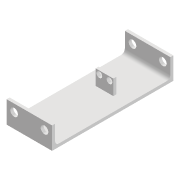
# Autodesk Inventor part: Top grip collecter grip
Saved by Autodesk Inventor 2020 (Build 240168000, 168)
## iProperties
Created: 2019-10-17
Part Number: Top grip collecter grip
Material: Generic
Document SubType Name: Modeling
Designer: ball
Density: 1 g/cm^3
Appearance: Default
Author: ball
Autodesk Inventor part; units mm, degrees
ref_plane "YZ Plane" through (0, 0, 0) normal (1, 0, 0) x (0, 1, 0)
ref_plane "XZ Plane" through (0, 0, 0) normal (0, 1, 0) x (-1, 0, 0)
sketch "Sketch1" plane through (0, 0, 0) normal (0, 1, 0) x (-1, 0, 0)
  line L0 (0, 0) -> (76.2, 0)
  line L1 (76.2, 0) -> (76.2, -203.2)
  line L2 (76.2, -203.2) -> (0, -203.2)
  line L3 (0, -203.2) -> (0, 0)
  dimension "d0" = 76.2
  dimension "d1" = 203.2
  constraints: 8 end point, 2 parallel, 1 horizontal, 1 perpendicular
  measures "d0" distance of L1.end L2.end
  measures "d1" distance of L0.end L1.end
extrude "Extrusion1" add sketch "Sketch1" along normal blind 36.83
sketch "Sketch2" plane through (-76.2, 0, 0) normal (0, 0, 1) x (1, 0, 0)
  circle A0 centre (63.5, 24.13) radius 6.4135
  circle A1 centre (12.7, 24.13) radius 6.4135
  line L0 (76.2, 0) -> (0, 0) projected
  line L1 (0, 0) -> (0, 36.83) projected
  dimension "d4" = 12.827
  dimension "d5" = 12.827
  dimension "d6" = 24.13
  dimension "d7" = 24.13
  dimension "d8" = 50.8
  dimension "d9" = 12.7
  constraints: 2 centre point
  measures "d4" diameter of A0
  measures "d5" diameter of A1
  measures "d6" distance from line of L0 A1.centre
  measures "d7" distance from line of L0 A0.centre
  measures "d8" distance of A0.centre A1.centre
  measures "d9" distance from line of L1 A1.centre
extrude "Extrusion2" cut sketch "Sketch2" against normal through all
sketch "Sketch3" plane through (0, 0, 0) normal (1, 0, 0) x (0, 0, -1)
  line L0 (0, 36.83) -> (203.2, 36.83) projected
  line L1 (5.08, 36.83) -> (198.12, 36.83)
  line L2 (198.12, 36.83) -> (198.12, 5.08)
  line L3 (198.12, 5.08) -> (5.08, 5.08)
  line L4 (5.08, 5.08) -> (5.08, 36.83)
  line L5 (0, 0) -> (0, 36.83) projected
  line L6 (203.2, 0) -> (203.2, 36.83) projected
  line L7 (203.2, 0) -> (0, 0) projected
  dimension "d12" = 5.08
  dimension "d13" = 5.08
  dimension "d14" = 5.08
  constraints: 8 end point, 2 parallel, 1 horizontal, 1 perpendicular, 1 point on line
  measures "d12" distance between parallel lines of L5 L4
  measures "d13" distance between parallel lines of L6 L2
  measures "d14" distance between parallel lines of L7 L3
extrude "Extrusion3" cut sketch "Sketch3" against normal through all contours L0 L2 L3 L4
fillet "Fillet1" radius 6.35 2 edges at (-38.1, 5.08, -198.12) (-38.1, 5.08, -5.08)
ref_plane "Work Plane1" through (-38.1, 0, 0) normal (1, 0, 0) x (0, 0, -1)
sketch "Sketch4" plane through (0, 5.08, -11.43) normal (0, 1, 0) x (1, 0, 0)
  line L0 (-60.3288, -11.303) -> (-60.3288, 191.643) construction
  line L1 (-15.4638, -11.303) -> (-15.4638, 191.643) construction
  line L2 (-23.0838, 119.2895) -> (-52.7088, 119.2895)
  line L3 (-52.7088, 114.2095) -> (-23.0838, 114.2095)
  line L4 (-52.7088, 114.2095) -> (-52.7088, 119.2895)
  line L5 (-23.0838, 114.2095) -> (-23.0838, 119.2895)
  line L6 (-24.257, 119.5032) -> (-34.9758, 119.5032) projected
  point P0 (0, -11.43)
  dimension "d19" = 7.62
  dimension "d20" = 7.62
  constraints: 10 end point, 2 perpendicular, 1 horizontal, 1 parallel, 1 vertical, 2 other
  measures "d19" distance between parallel lines of L0 L4
  measures "d20" distance between parallel lines of L1 L5
extrude "Extrusion4" add sketch "Sketch4" along normal blind 25.4
sketch "Sketch7" plane through (-52.7088, 5.08, -125.6395) normal (0, 0, 1) x (1, 0, 0)
  circle A0 centre (6.1541, 19.4644) radius 5.0173 construction
  circle A1 centre (6.1541, 19.4644) radius 4.826
  circle A2 centre (23.0924, 19.1199) radius 4.826
  circle A3 centre (23.0924, 19.462) radius 5.3594 projected
  circle A4 centre (6.1541, 19.8066) radius 5.3594 projected
  point P0 (52.7088, -5.08)
  dimension "d23" = 9.652
  dimension "d24" = 9.652
  constraints: 3 centre point, 1 coincident, 1 tangent
  measures "d23" diameter of A1
  measures "d24" diameter of A2
extrude "Extrusion5" cut sketch "Sketch7" against normal blind 6.35 contours A1 | A2
fillet "Fillet2" radius 3.175 4 edges at (-37.8963, 5.08, -125.6395) (-37.8963, 5.08, -130.7195) (-23.0838, 5.08, -128.1795) (-52.7088, 5.08, -128.1795)
sketch "Sketch8" plane through (0, 5.08, -11.43) normal (0, 1, 0) x (1, 0, 0)
  line L0 (-25.9664, 160.17) -> (-33.2664, 160.17) construction
  line L1 (-15.4638, -11.303) -> (-15.4638, 191.643) construction
  ellipse E0 centre (-46.5547, 158.3808) end of major axis (-51.9141, 158.3808) minor radius 0.1316 construction
  ellipse E1 centre (-46.5547, 161.5041) end of major axis (-51.3045, 161.5041) minor radius 0.1166 construction
  line L2 (-60.3288, -11.303) -> (-60.3288, 191.643) construction
  line L3 (-60.3288, -11.303) -> (-60.3288, 191.643) construction
  line L4 (-19.7164, 160.04) -> (-19.541, 180.14) construction
  line L5 (-19.7164, 160.04) -> (-19.541, 180.14) construction
  line L6 (-19.6387, 168.9455) -> (-19.673, 165.0128) construction
  line L7 (-19.6387, 168.9455) -> (-19.6387, 168.9455) construction
  line L8 (-19.6283, 170.1318) -> (-19.6387, 168.9455) construction
  line L9 (-19.6283, 170.1318) -> (-19.6283, 170.1318) construction
  line L10 (-19.6283, 170.1336) -> (-19.6283, 170.1318) construction
  line L11 (-19.6094, 172.2957) -> (-19.6283, 170.1336) construction
  line L12 (-19.6094, 172.2984) -> (-19.6094, 172.2957) construction
  line L13 (-19.6094, 172.2957) -> (-19.6094, 172.2984) construction
  line L14 (-19.6515, 167.4818) -> (-19.6094, 172.2957) construction
  line L15 (-19.6528, 167.3259) -> (-19.6515, 167.4818) construction
  line L16 (-19.6528, 167.3259) -> (-19.6528, 167.3259) construction
  line L17 (-19.6679, 165.5962) -> (-19.6528, 167.3259) construction
  line L18 (-19.6679, 165.5962) -> (-19.6679, 165.5962) construction
  line L19 (-19.653, 167.3096) -> (-19.6679, 165.5962) construction
  line L20 (-19.653, 167.3096) -> (-19.6494, 167.7197) construction
  line L21 (-19.6094, 172.2957) -> (-19.6494, 167.7197) construction
  line L22 (-19.6283, 170.1318) -> (-19.6094, 172.2957) construction
  line L23 (-19.6283, 170.1318) -> (-19.6283, 170.1318) construction
  line L24 (-19.6283, 170.13) -> (-19.6283, 170.1318) construction
  line L25 (-19.6717, 165.1614) -> (-19.6283, 170.13) construction
  line L26 (-19.6868, 163.4314) -> (-19.6717, 165.1614) construction
  line L27 (-19.6868, 163.4314) -> (-19.6868, 163.4314) construction
  line L28 (-19.673, 165.0128) -> (-19.6868, 163.4314) construction
  line L29 (-19.6094, 172.2957) -> (-19.6283, 170.1318) construction
  line L30 (-19.6094, 172.2957) -> (-19.6094, 172.2957) construction
  line L31 (-19.673, 165.0128) -> (-19.6094, 172.2957) construction
  line L32 (-19.6868, 163.4314) -> (-19.673, 165.0128) construction
  line L33 (-19.6868, 163.4314) -> (-19.6868, 163.4314) construction
  line L34 (-19.6868, 163.4334) -> (-19.6868, 163.4314) construction
  line L35 (-19.6679, 165.5962) -> (-19.6868, 163.4334) construction
  line L36 (-19.6679, 165.5962) -> (-19.6679, 165.5962) construction
  line L37 (-19.6679, 165.5979) -> (-19.6679, 165.5962) construction
  line L38 (-19.6552, 167.0544) -> (-19.6679, 165.5979) construction
  line L39 (-19.6552, 167.0544) -> (-19.6552, 167.0544) construction
  line L40 (-19.6411, 168.6735) -> (-19.6552, 167.0544) construction
  line L41 (-19.6411, 168.6735) -> (-19.6411, 168.6735) construction
  line L42 (-19.6283, 170.1318) -> (-19.6411, 168.6735) construction
  line L43 (-19.6283, 170.1318) -> (-19.6283, 170.1318) construction
  line L44 (-19.6868, 163.4314) -> (-19.6868, 163.4314) construction
  line L45 (-19.6094, 172.2957) -> (-19.6868, 163.4314) construction
  line L46 (-19.6868, 163.4314) -> (-19.6094, 172.2957) construction
  line L47 (-19.6868, 163.4314) -> (-19.6868, 163.4314) construction
  line L48 (-19.6472, 167.967) -> (-19.6868, 163.4314) construction
  line L49 (-19.6868, 163.4314) -> (-19.6472, 167.967) construction
  line L50 (-19.5888, 174.6572) -> (-19.584, 175.214) construction
  line L51 (-19.5788, 175.8099) -> (-19.5739, 176.3668) construction
  line L52 (-19.5858, 175.0075) -> (-19.5736, 176.4035) construction
  line L53 (-19.5736, 176.4035) -> (-19.5736, 176.4035) construction
  line L54 (-19.5736, 176.4035) -> (-19.5858, 175.0075) construction
  line L55 (-19.5858, 175.0075) -> (-19.5858, 175.0075) construction
  line L56 (-19.5858, 175.0075) -> (-19.5892, 174.6137) construction
  line L57 (-19.5892, 174.6137) -> (-19.5892, 174.6137) construction
  line L58 (-19.5892, 174.6137) -> (-19.5858, 175.0075) construction
  line L59 (-19.5858, 175.0075) -> (-19.5858, 175.0075) construction
  line L60 (-19.5844, 175.1679) -> (-19.5884, 174.7078) construction
  line L61 (-19.5831, 175.3099) -> (-19.5834, 175.2759) construction
  line L62 (-19.5789, 175.7906) -> (-19.5747, 176.2825) construction
  line L63 (-19.5781, 175.8923) -> (-19.5789, 175.7906) construction
  line L64 (-19.5736, 176.4035) -> (-19.58, 175.6688) construction
  line L65 (-19.5736, 176.4035) -> (-19.5736, 176.4035) construction
  line L66 (-19.5772, 175.9878) -> (-19.5736, 176.4035) construction
  line L67 (-19.5823, 175.4036) -> (-19.5772, 175.9878) construction
  line L68 (-19.5861, 174.9699) -> (-19.5861, 174.9699) construction
  line L69 (-19.5736, 176.4035) -> (-19.5861, 174.9699) construction
  line L70 (-19.5736, 176.4035) -> (-19.5736, 176.4035) construction
  line L71 (-19.5892, 174.6137) -> (-19.5736, 176.4035) construction
  line L72 (-19.5892, 174.6137) -> (-19.5892, 174.6137) construction
  line L73 (-19.5892, 174.6137) -> (-19.5892, 174.6137) construction
  line L74 (-19.5819, 175.4488) -> (-19.582, 175.4443) construction
  line L75 (-19.5736, 176.4035) -> (-19.5736, 176.4035) construction
  line L76 (-19.5892, 174.6137) -> (-19.5736, 176.4035) construction
  line L77 (-19.5892, 174.6137) -> (-19.5736, 176.4035) construction
  line L78 (-19.5736, 176.4035) -> (-19.5736, 176.4035) construction
  line L79 (-19.5736, 176.4035) -> (-19.5892, 174.6137) construction
  line L80 (-19.5892, 174.6137) -> (-19.5892, 174.6137) construction
  line L81 (-51.9141, 158.1619) -> (-51.9141, 159.0508) construction
  line L82 (0, 0) -> (-76.2, 0) construction
  line L83 (0, 180.34) -> (0, 0) construction
  line L84 (-76.2, 180.34) -> (0, 180.34) construction
  line L85 (-76.2, 0) -> (-76.2, 180.34) construction
  line L86 (-19.9088, 111.0345) -> (-19.9088, 122.4645) construction
  line L87 (-55.8838, 111.0345) -> (-19.9088, 111.0345) construction
  line L88 (-55.8838, 122.4645) -> (-55.8838, 111.0345) construction
  line L89 (-19.9088, 122.4645) -> (-55.8838, 122.4645) construction
  line L90 (-15.4638, 160.17) -> (-53.1828, 160.17) construction
  line L91 (-53.1828, 160.17) -> (-53.1828, 166.52) construction
  line L92 (-53.1828, 166.52) -> (-15.4638, 166.52) construction
  line L93 (-15.4638, 166.52) -> (-15.4638, 160.17) construction
  line L94 (-53.1828, 166.52) -> (-16.0988, 166.52)
  line L95 (-16.0988, 166.52) -> (-16.0988, 160.17)
  line L96 (-16.0988, 160.17) -> (-53.1828, 160.17)
  line L97 (-53.1828, 160.17) -> (-53.1828, 166.52)
  point P0 (0, -11.43)
  dimension "d28" = 37.719
  dimension "d29" = 6.35
  dimension "d30" = 37.084
  constraints: 22 end point, 4 parallel, 3 point on line, 3 vertical, 2 horizontal, 2 perpendicular, 6 other
  measures "d28" distance of L91.end L92.end
  measures "d29" distance of L90.end L91.end
  measures "d30" distance of L95.end L96.end
extrude "Extrusion6" add sketch "Sketch8" along normal blind 58.928
sketch "Sketch9" plane through (-53.1828, 5.08, -171.6) normal (0, 0, 1) x (1, 0, 0)
  line L0 (37.084, 0) -> (0, 0)
  line L1 (37.084, 0) -> (37.084, 58.928)
  line L2 (0, 58.928) -> (37.084, 58.928)
  line L3 (0, 0) -> (0, 58.928)
  ellipse E0 centre (12.3574, 19.462) end of major axis (12.3574, 179.2561) minor radius 1.3944 (13.7519, 19.462) -> (13.7293, 48.1267) ccw construction
  spline S0 degree 3 number of poles 88 construction
  line L4 (32.192, 49.4152) -> (14.9407, 49.4152) construction
  spline S1 degree 3 number of poles 79 construction
  ellipse E1 centre (34.7753, 19.462) end of major axis (34.7753, 179.2561) minor radius 1.3944 (33.4035, 48.1267) -> (33.3809, 19.462) ccw construction
  line L5 (32.1522, 9.6538) -> (14.9806, 9.6538) construction
  circle A0 centre (28.5664, 54.2513) radius 1.9685
  circle A1 centre (18.5664, 54.2513) radius 1.9685
  circle A2 centre (18.5664, 4.7532) radius 1.9685
  circle A3 centre (28.5664, 4.7532) radius 1.9685
  line L6 (33.4057, 49.4152) -> (13.7293, 49.4152) construction
  line L7 (13.7293, 49.4152) -> (13.7293, 9.6025) construction
  line L8 (13.7293, 9.6025) -> (33.4057, 9.6025) construction
  line L9 (33.4057, 9.6025) -> (33.4057, 49.4152) construction
  line L10 (12.7, 8.5732) -> (12.7, 50.4445)
  line L11 (12.7, 50.4445) -> (34.4349, 50.4445)
  line L12 (34.4349, 50.4445) -> (34.4349, 8.5732)
  line L13 (34.4349, 8.5732) -> (12.7, 8.5732)
  circle A4 centre (6.6281, 19.4449) radius 4.826
  circle A5 centre (6.6281, 19.8066) radius 3.175
  arc A6 (17.3164, 56.1354) -> (19.9164, 56.0646) centre (18.5664, 54.2646) ccw
  arc A7 (32.9664, 49.1464) -> (32.192, 49.4152) centre (32.192, 48.1652) ccw
  arc A8 (19.9164, 2.9646) -> (17.3164, 2.8938) centre (18.5664, 4.7646) ccw
  arc A9 (29.8164, 2.8938) -> (27.2164, 2.9646) centre (28.5664, 4.7646) ccw
  arc A10 (27.2164, 56.0646) -> (29.8164, 56.1354) centre (28.5664, 54.2646) ccw
  point P0 (53.1828, -5.08)
  dimension "d33" = 3.937
  dimension "d34" = 3.937
  dimension "d35" = 3.937
  dimension "d36" = 3.937
  dimension "d37" = 1.0293
  dimension "d38" = 9.652
  constraints: 16 end point, 5 centre point, 4 parallel, 2 perpendicular, 1 horizontal, 1 point on line, 5 other
  measures "d33" diameter of A0
  measures "d34" diameter of A1
  measures "d35" diameter of A2
  measures "d36" diameter of A3
  measures "d37" distance between parallel lines of L7 L10
  measures "d38" diameter of A4
extrude "Extrusion7" cut sketch "Sketch9" against normal up to surface (6.35 mm away) contours A0 | A1 | A2 | A3 | L10 L11 L12 L13 | A4 | A5
fillet "Fillet3" radius 3.175 3 edges at (-16.0988, 5.08, -174.775) (-34.6408, 5.08, -177.95) (-53.1828, 5.08, -174.775)
fillet "Fillet4" radius 2.54 1 edges at (-34.6408, 5.08, -171.6)
fillet "Fillet5" radius 3.175 12 edges at (-76.2, 36.83, -200.66) (0, 36.83, -200.66) (0, 36.83, -2.54) (-76.2, 36.83, -2.54) (-76.2, 18.415, 0) (0, 18.415, 0) (-76.2, 18.415, -203.2) (0, 18.415, -203.2) (-53.1828, 64.008, -174.775) (-16.0988, 64.008, -174.775) (-38.1, 36.83, -203.2) (-38.1, 36.83, 0)
fillet "Fillet6" radius 3.175 2 edges at (-52.7088, 30.48, -128.1795) (-23.0838, 30.48, -128.1795)
sketch "Sketch10" plane through (-35.7929, 8.255, -177.95) normal (0, 0, -1) x (-1, 0, 0)
  circle A0 centre (-11.1765, 51.0763) radius 1.9685 construction
  circle A1 centre (-11.1765, 51.0763) radius 4.6609 construction
  circle A2 centre (-1.1765, 51.0763) radius 1.9685 construction
  circle A3 centre (-1.1765, 51.0763) radius 4.6609 construction
  line L0 (-6.5156, 51.0763) -> (-8.8461, 47.0399)
  line L1 (-8.8461, 47.0399) -> (-13.507, 47.0399)
  line L2 (-13.507, 47.0399) -> (-15.8374, 51.0763)
  line L3 (-15.8374, 51.0763) -> (-13.507, 55.1128)
  line L4 (-13.507, 55.1128) -> (-8.8461, 55.1128)
  line L5 (-8.8461, 55.1128) -> (-6.5156, 51.0763)
  line L6 (3.4844, 51.0763) -> (1.1539, 47.0399)
  line L7 (1.1539, 47.0399) -> (-3.507, 47.0399)
  line L8 (-3.507, 47.0399) -> (-5.8374, 51.0763)
  line L9 (-5.8374, 51.0763) -> (-3.507, 55.1128)
  line L10 (-3.507, 55.1128) -> (1.1539, 55.1128)
  line L11 (1.1539, 55.1128) -> (3.4844, 51.0763)
  point P0 (-35.7929, -8.255)
  dimension "d45" = 9.3218
  dimension "d46" = 9.3218
  constraints: 24 end point, 4 coincident, 2 horizontal alignment, 30 other
extrude "Extrusion8" cut sketch "Sketch10" against normal blind 4.3688
body "Solid1"
